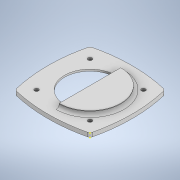
# Autodesk Inventor part: Boot Handle (Handle) Rev B
Saved by Autodesk Inventor 2021 (Build 250183000, 183)
## iProperties
Created: 2020-09-03
Part Number: Boot Handle (Handle) Rev B
Material: Generic
Document SubType Name: Modeling
Designer: cmzgt
Density: 1 g/cm^3
Appearance: Default
Author: cmzgt
## iProperties of the stored document _3DPrint.ipt
Created: 2021-06-28
Part Number: _3DPrint
Material: Generic
Document SubType Name: Modeling
Designer: cmzgt
Density: 1 g/cm^3
Appearance: Default
Author: cmzgt
Autodesk Inventor part; units mm, degrees
ref_plane "YZ Plane" through (0, 0, 0) normal (1, 0, 0) x (0, 1, 0)
ref_plane "XZ Plane" through (0, 0, 0) normal (0, 1, 0) x (-1, 0, 0)
ref_plane "XY Plane" through (0, 0, 0) normal (0, 0, 1) x (1, 0, 0)
sketch "Sketch1" plane through (0, 0, 0) normal (0, 1, 0) x (-1, 0, 0)
  line L0 (0, 0) -> (0, -71.12)
  line L1 (0, -71.12) -> (71.12, -71.12)
  line L2 (71.12, -71.12) -> (71.12, 0)
  line L3 (71.12, 0) -> (0, 0)
  arc A0 (71.12, -71.12) -> (71.12, 0) centre (-71.8439, -35.56) ccw
  arc A1 (0, 0) -> (0, -71.12) centre (142.9639, -35.56) ccw
  arc A2 (0, -71.12) -> (71.12, -71.12) centre (35.56, 71.8439) ccw
  arc A3 (71.12, 0) -> (0, 0) centre (35.56, -142.9639) ccw
  circle A4 centre (35.56, -35.56) radius 24.13
  dimension "d9" = 71.12
  dimension "d10" = 71.12
  dimension "d14" = 147.32
  dimension "d17" = 48.26
  dimension "d18" = 35.56
  dimension "d19" = 35.56
  constraints: 8 end point, 8 point on circle, 5 centre point, 3 equal radius, 3 perpendicular, 1 vertical
  measures "d9" distance of L0.start L0.end
  measures "d10" distance of L0.end L1.end
  measures "d14" radius of A3
  measures "d17" diameter of A4
  measures "d18" distance from line of A4.centre L0
  measures "d19" distance from line of A4.centre L1
extrude "Extrusion1" add sketch "Sketch1" along normal blind 3.81
fillet "Fillet1" radius 3.175 4 edges at (0, 1.905, 0) (0, 1.905, -71.12) (-71.12, 1.905, 0) (-71.12, 1.905, -71.12)
sketch "Sketch2" plane through (0, 3.81, 0) normal (0, 1, 0) x (1, 0, 0)
  point P0 (0, 0)
sketch "Sketch3" plane through (0, 0, 0) normal (0, -1, 0) x (1, 0, 0)
  circle A0 centre (-35.56, -35.56) radius 24.13 projected
  circle A1 centre (-35.56, -35.56) radius 31.75
  circle A2 centre (-35.56, -35.56) radius 24.13
  point P0 (0, 0)
  dimension "d23" = 63.5
  constraints: 2 centre point, 2 coincident
  measures "d23" diameter of A1
extrude "Extrusion2" cut sketch "Sketch3" against normal blind 2.1079
sketch "Sketch4" plane through (0, 0, 0) normal (0, -1, 0) x (1, 0, 0)
  circle A0 centre (-35.56, -35.56) radius 24.13 projected
  circle A1 centre (-35.56, -35.56) radius 31.75 projected
  circle A2 centre (-60.96, -10.16) radius 1.905
  arc A3 (-1.9053, 0.4605) -> (-69.2147, 0.4605) centre (-35.56, -142.9639) ccw construction
  line L0 (-35.56, 4.3561) -> (-35.56, -75.4761) construction
  arc A4 (-69.2147, -71.5805) -> (-1.9053, -71.5805) centre (-35.56, 71.8439) ccw construction
  arc A5 (-71.5805, -1.9053) -> (-71.5805, -69.2147) centre (71.8439, -35.56) ccw construction
  line L1 (-75.4761, -35.56) -> (4.3561, -35.56) construction
  arc A6 (0.4605, -69.2147) -> (0.4605, -1.9053) centre (-142.9639, -35.56) ccw construction
  line L2 (-75.4761, -35.56) -> (-75.4761, 1.4435) construction
  circle A7 centre (-10.16, -10.16) radius 1.905
  line L3 (4.3561, -35.56) -> (4.3561, 1.4435) construction
  circle A8 centre (-60.96, -60.96) radius 1.905
  circle A9 centre (-10.16, -60.96) radius 1.905
  point P0 (0, 0)
  dimension "d26" = 3.81
  dimension "d34" = 25.4
  dimension "d35" = 25.4
  dimension "d36" = 14.5161
  dimension "d37" = 14.5162
  dimension "d38" = 50.8
  dimension "d39" = 50.8
  constraints: 8 end point, 4 centre point, 4 point on circle, 3 symmetric about line, 3 vertical, 1 perpendicular, 1 tangent, 3 other
  measures "d26" diameter of A2
  measures "d34" distance from line of L0 A2.centre
  measures "d35" distance from line of L0 A7.centre
  measures "d36" distance from line of L2 A2.centre
  measures "d37" distance from line of L3 A7.centre
  measures "d38" distance of A2.centre A8.centre
  measures "d39" distance of A9.centre A7.centre
extrude "Extrusion3" cut sketch "Sketch4" against normal blind 25.4 contours A2 | A7 | A8 | A9
sketch "Sketch6" plane through (0, 0, 0) normal (0, -1, 0) x (1, 0, 0)
  point P0 (0, 0)
sketch "Sketch8" plane through (0, 3.81, 0) normal (0, 1, 0) x (1, 0, 0)
  circle A0 centre (-35.56, 35.56) radius 24.13 projected
  circle A1 centre (-35.56, 35.56) radius 24.13 construction
  line L0 (-35.56, 59.69) -> (-35.56, 64.77) construction
  line L1 (-35.56, 11.43) -> (-35.56, 6.35) construction
  line L2 (-11.43, 35.56) -> (-6.35, 35.56) construction
  arc A2 (-35.56, 6.35) -> (-35.56, 64.77) centre (-35.56, 35.56) ccw
  line L3 (-35.56, 64.77) -> (-35.56, 6.35)
  point P0 (0, 0)
  dimension "d44" = 5.08
  dimension "d45" = 5.08
  dimension "d46" = 5.08
  constraints: 8 end point, 6 point on circle, 3 vertical, 1 centre point, 1 horizontal
  measures "d44" distance of L0.start L0.end
  measures "d45" distance of L1.start L1.end
  measures "d46" distance of L2.start L2.end
extrude "Extrusion5" add sketch "Sketch8" along normal blind 3.556 contours A0 L3 | A0 L3 A2 picked at (-27.7183, 37.3498)
fillet "Fillet2" radius 3.048 1 edges at (-6.35, 3.81, -35.56)
body "Solid1"
